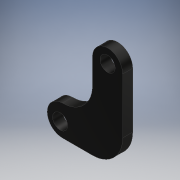
# Autodesk Inventor part: EE Link
Saved by Autodesk Inventor 2017 (Build 210142000, 142)
## iProperties
Created: 2018-10-18
Part Number: EE Link
Material: Generic
Document SubType Name: Modeling
Designer: Cameron
Density: 1 g/cm^3
Appearance: Glossy - Black
Author: Cameron
Autodesk Inventor part; units mm, degrees
ref_plane "YZ Plane" through (0, 0, 0) normal (1, 0, 0) x (0, 1, 0)
ref_plane "XZ Plane" through (0, 0, 0) normal (0, 1, 0) x (-1, 0, 0)
ref_plane "XY Plane" through (0, 0, 0) normal (0, 0, 1) x (1, 0, 0)
sketch "Sketch1" plane through (0, 0, 0) normal (0, 1, 0) x (-1, 0, 0)
  line L0 (3, 0) -> (3, 0)
  line L1 (15, -17) -> (15, -17)
  line L2 (12, -20) -> (6, -20)
  line L3 (0, -14) -> (0, -3)
  line L4 (12, -14) -> (12, -14)
  line L5 (6, -3) -> (6, -8)
  arc A0 (15, -17) -> (12, -14) centre (12, -17) ccw
  arc A1 (12, -20) -> (15, -17) centre (12, -17) ccw
  arc A2 (6, -3) -> (3, 0) centre (3, -3) ccw
  arc A3 (3, 0) -> (0, -3) centre (3, -3) ccw
  arc A4 (6, -8) -> (12, -14) centre (12, -8) ccw
  arc A5 (0, -14) -> (6, -20) centre (6, -14) ccw
  circle A6 centre (3, -2.7294) radius 1.5
  circle A7 centre (12.4501, -17.3795) radius 1.5
  point P0 (0, 0)
  point P1 (15, -20)
  point P2 (15, 0)
  point P3 (0, -20)
  dimension "d0" = 15
  dimension "d1" = 20
  dimension "d2" = 6
  dimension "d3" = 3
  dimension "d4" = 6
  dimension "d5" = 3
  dimension "d6" = 3
  constraints: 12 end point, 12 point on circle, 12 tangent, 8 centre point, 8 point on line, 4 equal radius, 2 parallel, 1 horizontal, 1 perpendicular
  measures "d0" distance of point (15, -20) point (0, -20)
  measures "d1" distance of point (15, 0) point (15, -20)
  measures "d2" distance between parallel lines of L2 L4
  measures "d3" radius of A0
  measures "d4" radius of A4
  measures "d5" diameter of A6
  measures "d6" diameter of A7
extrude "Extrusion1" add sketch "Sketch1" along normal blind 2
body "Solid1"
